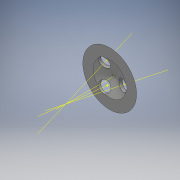
# Autodesk Inventor part: Splitter
Saved by Autodesk Inventor 2016 (Build 200138000, 138)
## iProperties
Created: 2016-01-21
Part Number: Splitter
Material: Generic
Document SubType Name: Modeling
Designer: KA ROSIE
Density: 1 g/cm^3
Appearance: Default
Author: KA ROSIE
Autodesk Inventor part; units mm, degrees
ref_plane "YZ Plane" through (0, 0, 0) normal (1, 0, 0) x (0, 1, 0)
ref_plane "XZ Plane" through (0, 0, 0) normal (0, 1, 0) x (-1, 0, 0)
sketch "Sketch1" plane through (0, 0, 0) normal (0, 0, 1) x (1, 0, 0)
  line L0 (0, -0.2679) -> (0, 1.6077) projected
  line L1 (3.0681, 0) -> (5, 0)
  line L2 (5, 0) -> (0.3349, 1.25)
  line L3 (0, 1.3397) -> (0, 0)
  line L4 (0, 0) -> (0.3349, 1.25) construction
  line L5 (0, 0) -> (1.2941, 0) construction
  line L6 (0.3349, 1.25) -> (0.2055, 0.767)
  line L7 (0.2055, 0.767) -> (3.0681, 0)
  dimension "d2" = 5
  dimension "d3" = 15
  dimension "d4" = 75
  dimension "d16" = 0.5
  constraints: 14 end point, 2 horizontal, 2 point on line, 1 collinear, 1 equal length, 1 parallel
  measures "d2" distance of L3.end L1.end
  measures "d3" angle of L2 L1
  measures "d4" angle of L5 L4
  measures "d16" distance of L2.end L6.end
revolve "Revolution1" add sketch "Sketch1" angle 360 about axis through (0, -10, 0) along (0, 1, 0)
ref_plane "Work Plane2" through (5, 0, 0) normal (0.2588, 0.9659, 0) x (-0.9659, 0.2588, 0)
sketch "Sketch5" plane through (5, 0, 0) normal (0.2588, 0.9659, 0) x (-0.9659, 0.2588, 0)
  circle A0 centre (2.7092, 0) radius 1
  point P0 (4.8296, 0)
  dimension "d18" = 2
  constraints: 1 centre point
  measures "d18" diameter of A0
extrude "Extrusion2" cut sketch "Sketch5" against normal through all
pattern_circular "Circular Pattern3" count 3 over 360 about axis through (0, -10, 0) along (0, 1, 0) of "Extrusion2"
body "Solid2"
